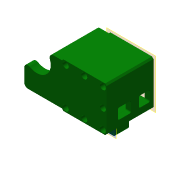
# Autodesk Inventor part: cellSTORM_v5_cellphonestage
Saved by Autodesk Inventor 2022 (Build 260153000, 153)
## iProperties
Created: 2020-04-25
Part Number: cellSTORM_v5_cellphonestage
Material: Generic
Document SubType Name: Modeling
Designer: diederichbenedict
Density: 1 g/cm^3
Appearance: Dark Green
Author: diederichbenedict
Autodesk Inventor part; units mm, degrees
ref_plane "YZ Plane" through (0, 0, 0) normal (1, 0, 0) x (0, 1, 0)
ref_plane "XZ Plane" through (0, 0, 0) normal (0, 1, 0) x (-1, 0, 0)
ref_plane "XY Plane" through (0, 0, 0) normal (0, 0, 1) x (1, 0, 0)
ref_plane "Work Plane1" through (0, 0, 0) normal (0, 0, 1) x (1, 0, 0)
ref_plane "Arbeitsebene4" through (-45, -22, 45) normal (0, 0, -1) x (0, 1, 0)
sketch "Sketch1" plane through (0, 0, 0) normal (0, 0, 1) x (1, 0, 0)
  circle A0 centre (25, 25) radius 1.95 projected
  circle A1 centre (25, 0) radius 1.95 projected
  circle A2 centre (0, 25) radius 1.95 projected
  circle A3 centre (-25, 0) radius 1.95 projected
  circle A4 centre (-25, -25) radius 1.95 projected
  circle A5 centre (25, 25) radius 1.95 projected
  circle A6 centre (25, -25) radius 1.95 projected
  circle A7 centre (-25, 25) radius 1.95 projected
  circle A8 centre (25, 0) radius 1.95 projected
  circle A9 centre (0, -25) radius 1.95 projected
  line L0 (-28, 30) -> (-30, 28) projected
  line L1 (-30, 28) -> (-30, -28) projected
  line L2 (-30, -28) -> (-28, -30) projected
  line L3 (-28, -30) -> (28, -30) projected
  line L4 (28, -30) -> (30, -28) projected
  line L5 (30, -28) -> (30, 28) projected
  line L6 (30, 28) -> (28, 30) projected
  line L7 (28, 30) -> (-28, 30) projected
  point P0 (0, 0)
extrude "Extrusion1" add sketch "Sketch1" along normal up to surface (45 mm away)
sketch "Sketch3" plane through (-30, -28, 0) normal (-1, 0, 0) x (0, 0, 1)
  line L0 (0, 56) -> (0, 0) projected
  line L1 (0, 0) -> (45, 0) projected
  line L2 (0, 56) -> (45, 56) projected
  line L3 (45, 56) -> (45, 0) projected
  point P0 (0, 28)
extrude "Extrusion3" add sketch "Sketch3" along normal blind 10
sketch "Sketch4" plane through (22, -22, 0) normal (0, 0, 1) x (1, 0, 0)
  circle A0 centre (-22, -3) radius 1.95 projected
  circle A1 centre (-47, 47) radius 1.95 projected
  circle A2 centre (3, -3) radius 1.95 projected
  circle A3 centre (-47, -3) radius 1.95 projected
  circle A4 centre (-47, 22) radius 1.95 projected
  circle A5 centre (-22, 47) radius 1.95 projected
  circle A6 centre (3, 22) radius 1.95 projected
  circle A7 centre (3, 47) radius 1.95 projected
  line L0 (-50, 52) -> (-52, 50) projected
  line L1 (6, 52) -> (-50, 52) projected
  line L2 (8, 50) -> (6, 52) projected
  line L3 (8, -6) -> (8, 50) projected
  line L4 (6, -8) -> (8, -6) projected
  line L5 (-50, -8) -> (6, -8) projected
  line L6 (-52, -6) -> (-50, -8) projected
  line L7 (-52, -6) -> (-62, -6) projected
  line L8 (-62, 50) -> (-62, -6) projected
  line L9 (-52, 50) -> (-62, 50) projected
  line L10 (-45.05, 45.05) -> (1.05, 45.05)
  line L11 (1.05, 45.05) -> (1.05, -1.05)
  line L12 (1.05, -1.05) -> (-45.05, -1.05)
  line L13 (-45.05, -1.05) -> (-45.05, 45.05)
  circle A8 centre (-47, 22) radius 1.95 projected
  line L14 (-45.05, 0) -> (-59, 0)
  line L15 (-59, 0) -> (-59, 44)
  line L16 (-59, 44) -> (-45.05, 44)
  line L17 (-45.05, 44) -> (-45.05, 0)
  point P0 (-45.05, 22)
  dimension "d55" = 6
  dimension "d56" = 6
  dimension "d57" = 3
  constraints: 16 end point, 4 parallel, 3 tangent, 2 horizontal, 2 perpendicular, 1 point on line
  measures "d55" distance between parallel lines of L14 L7
  measures "d56" distance between parallel lines of L9 L16
  measures "d57" distance between parallel lines of L15 L8
extrude "Extrusion4" cut sketch "Sketch4" along normal through all contours L12 L13 L10 L11 | L14 L15 L16 L13
sketch "Sketch6" plane through (-40, -28, 0) normal (-1, 0, 0) x (0, 0, 1)
  line L0 (0, 56) -> (0, 0) projected
  line L1 (0, 0) -> (45, 0) projected
  line L2 (45, 56) -> (0, 56) projected
  line L3 (45, 0) -> (45, 56) projected
  point P0 (0, 28)
extrude "Extrusion6" add sketch "Sketch6" along normal blind 5
sketch "Sketch7" plane through (-45, -28, 0) normal (-1, 0, 0) x (0, 0, 1)
  circle A0 centre (41, 25.7717) radius 1.45 projected
  circle A1 centre (23.9, 21.2512) radius 1.45 projected
  circle A2 centre (3.3174, 32.2512) radius 1.45 projected
  circle A3 centre (3.3174, 53) radius 1.45 projected
  line L0 (40, 45) -> (40, 11) projected
  circle A4 centre (41, 8.1883) radius 1.45 projected
  circle A5 centre (4.9143, 21.2512) radius 1.45 projected
  circle A6 centre (23.9337, 3.5995) radius 1.45 projected
  circle A7 centre (41, 25.7717) radius 1.45 projected
  circle A8 centre (41.0502, 56) radius 1.45 projected
  circle A9 centre (41, 0.7395) radius 1.45 projected
  circle A10 centre (23.9, 21.2512) radius 1.45 projected
  circle A11 centre (23.9, 13.4229) radius 1.45 projected
  circle A12 centre (41, 43.0063) radius 1.45 projected
  line L1 (37.1004, -11.7636) -> (45, -11.7636) projected
  line L2 (45, -11.7636) -> (45, 58) projected
  line L3 (26.9, 58) -> (26.9, 25.2512) projected
  line L4 (26.9, 25.2512) -> (-10.2763, 25.2512) projected
  line L5 (-10.2763, 25.2512) -> (37.1004, -11.7636) projected
  line L6 (45, 58) -> (26.9, 58) projected
  point P0 (0, 28)
  point P1 (4.6577, 21.4172)
hole "Hole1" at (-45, 15.0063, 41) at (-45, -2.2283, 41) at (-45, -19.8117, 41) at (-45, -14.5771, 23.9) at (-45, -6.7488, 23.9) at (-45, 4.2512, 3.3174) at (-45, 25, 3.3174) at (-45, -6.7488, 4.9143) direction (1, 0, 0) diameter 2.9 depth 20 tip angle 118
ref_plane "Arbeitsebene3" through (-16.8987, -56.0499, 18.5) normal (0, 0, -1) x (1, 0, 0)
sketch "Skizze8" plane through (-16.8987, -56.0499, 18.5) normal (0, 0, -1) x (1, 0, 0)
  line L0 (-11.7173, -14.1596) -> (11.2824, -14.2743) projected
  line L1 (-11.7173, -14.1596) -> (11.2824, -14.2743) projected
  circle A0 centre (11.4094, 11.2112) radius 1.025 projected
  arc A1 (13.9094, 11.1987) -> (11.4218, 13.7112) centre (11.4094, 11.2112) ccw projected
  circle A2 centre (11.2948, -11.7885) radius 1.025 projected
  line L2 (13.9094, 11.1987) -> (13.7947, -11.801) projected
  arc A3 (13.9094, 11.1987) -> (11.4218, 13.7112) centre (11.4094, 11.2112) ccw projected
  line L3 (-11.5779, 13.8258) -> (11.4218, 13.7112) projected
  arc A4 (-11.5779, 13.8258) -> (-14.0903, 11.3383) centre (-11.5903, 11.3258) ccw projected
  line L4 (-14.2049, -11.6614) -> (-14.0903, 11.3383) projected
  arc A5 (-14.2049, -11.6614) -> (-11.7174, -14.1739) centre (-11.7049, -11.6739) ccw projected
  line L5 (11.2823, -14.2885) -> (-11.7174, -14.1739) projected
  arc A6 (11.2823, -14.2885) -> (13.7947, -11.801) centre (11.2948, -11.7885) ccw projected
  circle A7 centre (-0.1478, -0.2313) radius 11 projected
  circle A8 centre (-11.5903, 11.3258) radius 1.025 projected
  circle A9 centre (11.4094, 11.2112) radius 1.025 projected
  circle A10 centre (11.2948, -11.7885) radius 1.025 projected
  circle A11 centre (-11.7049, -11.6739) radius 1.025 projected
  line L6 (38.8987, -34.0499) -> (-28.1013, -34.0499) projected
  line L7 (38.8987, -34.0499) -> (-28.1013, -34.0499) projected
  line L8 (-14, -14) -> (13.7838, -14)
  line L9 (13.7838, -14) -> (13.7838, -34.0499)
  line L10 (13.7838, -34.0499) -> (-14, -34.0499)
  line L11 (-14, -34.0499) -> (-14, -14)
  line L12 (-14, -14) -> (-28.1013, -34.0499)
  line L13 (38.8987, -34.0499) -> (-28.1013, -34.0499) projected
  line L14 (-14, -34.0499) -> (-28.1013, -34.0499)
  line L15 (-28.1013, -34.0499) -> (-14, -14)
  line L16 (-14, -14) -> (-14.1998, -10.6365)
  line L17 (13.7838, -14) -> (13.7947, -11.801)
  point P0 (16.8987, -56.0499)
  constraints: 18 end point, 3 collinear, 2 parallel, 2 point on line, 1 horizontal, 1 perpendicular
extrude "Extrusion7" add sketch "Skizze8" along normal up to surface (18.5 mm away) contours L2 A6 L8 A5 L16 L4 A4 L3 A1 | L17 L8 A6 | L8 L9 L6 L11 A5 L5 A6 | A6 L5 A5 L8 | L8 L16 A5 | L11 L6 L12
sketch "Skizze12" plane through (-28, 30, 45) normal (0, 0, 1) x (1, 0, 0)
  line L0 (56, 0) -> (0, 0) projected
  line L1 (0, 0) -> (-2, -2) projected
  line L2 (-2, -2) -> (-17, -2) projected
  line L3 (-17, -58) -> (-17, -2) projected
  line L4 (-2, -58) -> (-17, -58) projected
  line L5 (-2, -58) -> (0, -60) projected
  line L6 (0, -60) -> (56, -60) projected
  line L7 (56, -60) -> (58, -58) projected
  line L8 (58, -58) -> (58, -2) projected
  line L9 (58, -2) -> (56, 0) projected
  circle A0 centre (53, -5) radius 1.95 projected
  circle A1 centre (53, -30) radius 1.95 projected
  circle A2 centre (28, -5) radius 1.95 projected
  circle A3 centre (3, -55) radius 1.95 projected
  circle A4 centre (53, -55) radius 1.95 projected
  circle A5 centre (3, -5) radius 1.95 projected
  circle A6 centre (28, -55) radius 1.95 projected
  circle A7 centre (45, -13) radius 3.5 construction
  circle A8 centre (-12, -47) radius 3.5 construction
  circle A9 centre (-12, -13) radius 3.5 construction
  circle A10 centre (45, -47) radius 3.5 construction
  line L10 (50, -52) -> (50, -8) construction
  line L11 (50, -8) -> (-18.5637, -8) construction
  arc A11 (-40, -33.2922) -> (-18.5637, -8) centre (-35.65, -15.2488) ccw construction
  line L12 (-40, -33.2922) -> (-40, -52) construction
  line L13 (-40, -52) -> (50, -52) construction
  circle A12 centre (-35.65, -15.2488) radius 18.5603
  line L14 (-17, -2) -> (-22.6518, -2)
  line L15 (-52.6465, -22.7056) -> (-52.6465, -58)
  line L16 (-52.6465, -58) -> (-17, -58)
  line L17 (28, -53.05) -> (4.95, -53.05) projected
  line L18 (4.95, -53.05) -> (4.95, -52) projected
  line L19 (4.95, -8) -> (4.95, -6.95) projected
  line L20 (4.95, -6.95) -> (28, -6.95) projected
  line L21 (28, -6.95) -> (51.05, -6.95) projected
  line L22 (51.05, -6.95) -> (51.05, -30) projected
  line L23 (51.05, -30) -> (51.05, -53.05) projected
  line L24 (51.05, -53.05) -> (28, -53.05) projected
  line L25 (4.95, -52) -> (-9, -52) projected
  line L26 (-9, -52) -> (-9, -8) projected
  line L27 (-9, -8) -> (4.95, -8) projected
  point P0 (28, -30)
  constraints: 6 end point, 3 point on circle, 2 vertical alignment, 1 centre point, 1 coincident, 1 collinear, 1 horizontal, 1 horizontal alignment, 1 perpendicular, 1 vertical
ref_plane "Arbeitsebene5" through (-68, -22, 63) normal (0, 0, 1) x (1, 0, 0)
extrude "Extrusion10" add sketch "Skizze12" along normal up to surface (18 mm away) contours L9 L8 L7 L6 L5 L4 L3 L2 L1 L0 | L3 L16 L15 A12 L14 | L23 L24 L17 L18 L25 L26 L27 L19 L20 L21 L22
fillet "Rundung1" radius 5 3 edges at (-50.6518, 28, 54) (-80.6465, 7.2944, 54) (-80.6465, -28, 54)
sketch "Skizze13" plane through (-40.7801, -28, 18.5) normal (0, -1, 0) x (1, 0, 0)
  line L0 (-34.8664, 26.5) -> (-39.8664, 26.5) projected
  line L1 (-1.2199, 29.7426) -> (-3.6199, 32.1426) projected
  line L2 (-34.8664, 26.5) -> (-34.8664, 44.5) projected
  line L3 (-34.8664, 26.5) -> (-4.2199, 26.5) projected
  line L4 (-4.2199, -18.5) -> (-4.2199, 26.5) projected
  line L5 (0, -18.5) -> (-4.2199, -18.5) projected
  line L6 (0, -18.5) -> (0, 0) projected
  line L7 (0, 0) -> (10.7801, 0) projected
  line L8 (10.7801, 0) -> (10.7801, 44.5) projected
  line L9 (10.7801, 44.5) -> (-34.8664, 44.5) projected
  line L10 (-4.2199, 26.5) -> (-11.2909, 33.5711)
  line L11 (-4.2199, 26.5) -> (5.7801, 26.5) construction
  line L12 (-11.2909, 33.5711) -> (-39.8664, 33.5711)
  line L13 (-39.8664, 44.5) -> (-39.8664, 26.5) projected
  line L14 (-39.8664, 26.5) -> (-4.2199, 26.5)
  point P0 (40.7801, -18.5)
  point P1 (-34.8664, 26.5)
  dimension "d44" = 10
  dimension "d45" = 135
  constraints: 8 end point, 2 horizontal, 1 equal length, 1 parallel, 1 point on line
  measures "d44" distance of L3.end L10.end
  measures "d45" angle of L11 L10
extrude "Extrusion11" cut sketch "Skizze13" against normal through all contours L0 L13 L12 L2 | L2 L12 L10 L3
sketch "Skizze14" plane through (-28, -30, 63) normal (0, 0, 1) x (1, 0, 0)
  arc A0 (-52.6465, 7) -> (-47.6465, 2) centre (-47.6465, 7) ccw projected
  line L0 (-2, 2) -> (-47.6465, 2) projected
  line L1 (0, 0) -> (-2, 2) projected
  line L2 (56, 0) -> (0, 0) projected
  line L3 (58, 2) -> (56, 0) projected
  line L4 (58, 58) -> (58, 2) projected
  line L5 (56, 60) -> (58, 58) projected
  line L6 (0, 60) -> (56, 60) projected
  line L7 (-2, 58) -> (0, 60) projected
  line L8 (-13.5809, 58) -> (-2, 58) projected
  arc A1 (-13.5809, 58) -> (-18.2644, 51.2494) centre (-13.5809, 53) ccw projected
  arc A2 (-45.1006, 28.7771) -> (-18.2644, 51.2494) centre (-35.65, 44.7512) ccw projected
  arc A3 (-45.1006, 28.7771) -> (-52.6465, 24.4738) centre (-47.6465, 24.4738) ccw projected
  line L9 (-52.6465, 7) -> (-52.6465, 24.4738) projected
  circle A4 centre (28, 5) radius 1.95 projected
  circle A5 centre (3, 55) radius 1.95 projected
  circle A6 centre (53, 5) radius 1.95 projected
  circle A7 centre (3, 5) radius 1.95 projected
  circle A8 centre (28, 55) radius 1.95 projected
  circle A9 centre (53, 30) radius 1.95 projected
  circle A10 centre (53, 55) radius 1.95 projected
  point P0 (28, 30)
hole "Bohrung3" at (-25, -25, 63) at (0, -25, 63) at (25, -25, 63) at (25, 0, 63) at (25, 25, 63) at (0, 25, 63) at (-25, 25, 63) direction (0, 0, -1) diameter 4.5 depth 60 tip angle 118 counterbore diameter 8 counterbore depth 55
sketch "Skizze15" plane through (30, -28, 0) normal (1, 0, 0) x (0, 0, -1)
  line L0 (-47.8868, 8.469) -> (-30.273, 8.469)
  line L1 (-30.273, 8.469) -> (-30.273, 22.7633)
  line L2 (-30.273, 22.7633) -> (-47.8868, 22.7633)
  line L3 (-47.8868, 22.7633) -> (-47.8868, 8.469)
  circle A0 centre (-4.9143, 21.2512) radius 1.45 projected
  line L4 (-19.6369, 8.469) -> (-4.9143, 8.469)
  line L5 (-4.9143, 8.469) -> (-4.9143, 22.7012)
  line L6 (-4.9143, 22.7012) -> (-19.6369, 22.7012)
  line L7 (-19.6369, 22.7012) -> (-19.6369, 8.469)
  point P0 (0, 28)
  point P1 (-4.9143, 19.8012)
  constraints: 16 end point, 4 parallel, 2 horizontal, 2 perpendicular, 1 point on line, 2 other
extrude "Extrusion12" cut sketch "Skizze15" against normal blind 10 contours L3 L2 L1 L0 | L5 A0 | A0 L5 L4 L7 L6 picked at (-5.3505, 21.627)
fillet "Rundung2" radius 2 9 edges at (26.525, -19.531, 30.273) (25, -19.531, 47.8868) (26.525, -5.2367, 30.273) (25, -5.2367, 47.8868) (26.525, -5.2988, 19.6369) (21.5075, -23.05, 26.5) (26.525, -19.531, 19.6369) (26.525, -19.531, 4.9143) (26.525, -5.2988, 4.9143)
body "Solid1"
